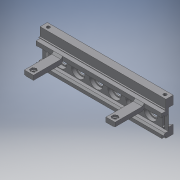
# Autodesk Inventor part: Case_top_back
Saved by Autodesk Inventor 2016 SP2 (Build 200236200, 236)
## iProperties
Created: 2018-06-26
Part Number: Case_top_back
Material: Generisch
Document SubType Name: Modeling
Designer: Nils
Density: 1 g/cm^3
Appearance: Vorgabe
Author: Nils
Autodesk Inventor part; units mm, degrees
ref_plane "YZ Plane" through (0, 0, 0) normal (1, 0, 0) x (0, 1, 0)
ref_plane "XZ Plane" through (0, 0, 0) normal (0, 1, 0) x (-1, 0, 0)
ref_plane "XY Plane" through (0, 0, 0) normal (0, 0, 1) x (1, 0, 0)
sketch "Skizze1" plane through (0, 0, 0) normal (1, 0, 0) x (0, 1, 0)
  line L0 (14.121, -6.5137) -> (22.121, -6.5137) projected
  line L1 (14.121, -15.8137) -> (14.121, -6.5137) projected
  line L2 (22.121, -6.5137) -> (22.121, -15.9372) projected
  line L3 (22.121, -34.3902) -> (22.121, -43.8137) projected
  line L4 (22.121, -43.8137) -> (14.121, -43.8137) projected
  line L5 (14.121, -38.3137) -> (14.121, -43.8137) projected
  line L6 (12.621, -15.8137) -> (14.121, -15.8137) projected
  line L7 (12.621, -15.8137) -> (12.621, -16.3137) projected
  line L8 (14.121, -17.8137) -> (12.621, -16.3137) projected
  line L9 (22.121, -15.9372) -> (22.121, -34.3902)
  line L10 (14.121, -43.8137) -> (14.121, -41.8137)
  line L11 (14.121, -41.8137) -> (9.621, -41.8137)
  line L12 (9.621, -41.8137) -> (9.621, -38.3137)
  line L13 (9.621, -38.3137) -> (11.421, -40.1137)
  line L14 (11.421, -40.1137) -> (13.221, -38.3137)
  line L15 (13.221, -38.3137) -> (16.691, -38.3137)
  line L16 (16.691, -38.3137) -> (16.691, -22.3437)
  line L17 (16.691, -22.3437) -> (13.221, -22.3437)
  line L18 (13.221, -22.3437) -> (11.421, -20.5437)
  line L19 (13.221, -22.3437) -> (15.7666, -22.3437) construction
  line L20 (11.421, -20.5437) -> (9.621, -22.3437)
  line L21 (9.621, -22.3437) -> (9.621, -17.8137)
  line L22 (9.621, -17.8137) -> (14.121, -17.8137)
  point P0 (0, 0)
  dimension "d0" = 2
  dimension "d1" = 4.5
  dimension "d2" = 3.5
  dimension "d3" = 3.47
  dimension "d4" = 15.97
  dimension "d5" = 1.8
  dimension "d6" = 45
  dimension "d7" = 135
  dimension "d8" = 4.53
  dimension "d9" = 1.8
  dimension "d10" = 4.5
  constraints: 28 end point, 7 perpendicular, 2 equal length, 2 vertical, 1 horizontal, 1 parallel, 1 point on line
  measures "d0" distance of L4.end L10.end
  measures "d1" distance of L10.end L11.end
  measures "d2" distance of L11.end L12.end
  measures "d3" distance of L14.end L15.end
  measures "d4" distance of L15.end L16.end
  measures "d5" horizontal distance of L12.end L13.end
  measures "d6" angle of L13 L12
  measures "d7" angle of L19 L18
  measures "d8" distance of L20.end L21.end
  measures "d9" horizontal distance of L18.end L17.end
  measures "d10" distance of L21.end L8.start
extrude "Extrusion1" add sketch "Skizze1" along normal blind 69.4
sketch "Skizze2" plane through (0, 22.121, -6.5137) normal (0, 1, 0) x (1, 0, 0)
  line L0 (128.7, 33.8232) -> (128.7, 3.4768) projected
  line L1 (0, 0) -> (138.8, 0) projected
  line L2 (10.1, 3.4768) -> (10.1, 33.8232) projected
  line L3 (0, 37.3) -> (138.8, 37.3) projected
  line L4 (0, 9.308) -> (0, 27.992)
  line L5 (0, 37.3) -> (0, 0) projected
  line L6 (138.8, 27.992) -> (128.7, 33.8232) projected
  line L7 (128.7, 3.4768) -> (138.8, 9.308) projected
  line L8 (138.8, 0) -> (138.8, 9.308) projected
  line L9 (0, 0) -> (0, 9.308) projected
  line L10 (0, 9.308) -> (10.1, 3.4768) projected
  line L11 (10.1, 33.8232) -> (0, 27.992) projected
  line L12 (0, 27.992) -> (0, 37.3) projected
  line L13 (138.8, 27.992) -> (138.8, 37.3) projected
  point P0 (0, -6.5137)
  constraints: 2 end point, 1 collinear
extrude "Extrusion2" cut sketch "Skizze2" against normal blind 5 contours L11 L2 L10 L4
sketch "Skizze3" plane through (0, 9.621, -22.3437) normal (0, -1, 0) x (1, 0, 0)
  line L0 (19.4, 2.53) -> (29.4, 2.53) projected
  line L1 (29.4, 2.53) -> (29.4, -2.47) projected
  line L2 (29.4, -2.47) -> (19.4, -2.47) projected
  line L3 (19.4, -2.47) -> (19.4, 2.53) projected
  point P0 (0, 22.3437)
extrude "Extrusion3" add sketch "Skizze3" along normal blind 32.25
chamfer "Fase1" distance 2.4 angle 45 1 edges at (24.4, 9.621, -24.8137)
chamfer "Fase2" distance 2 angle 45 1 edges at (24.4, 9.621, -19.8137)
sketch "Skizze4" plane through (29.4, -22.629, -24.8137) normal (0, 0, -1) x (-1, 0, 0)
  circle A0 centre (5, 5) radius 1.75
  line L0 (0, 0) -> (10, 0) projected
  line L1 (10, 30.25) -> (10, 0) projected
  point P0 (29.4, 22.629)
  point P1 (10, 32.25)
  dimension "d23" = 3.5
  dimension "d24" = 5
  dimension "d25" = 5
  constraints: 1 centre point
  measures "d23" diameter of A0
  measures "d24" distance from line of L0 A0.centre
  measures "d25" distance from line of L1 A0.centre
extrude "Extrusion4" cut sketch "Skizze4" against normal blind 32.25
sketch "Skizze6" plane through (0, 14.121, -6.5137) normal (0, 0, 1) x (1, 0, 0)
  circle A0 centre (5, 4) radius 1.75 projected
  point P0 (0, -14.121)
extrude "Extrusion5" cut sketch "Skizze6" against normal blind 34.75
sketch "Skizze7" plane through (0, 9.621, -22.3437) normal (0, -1, 0) x (1, 0, 0)
  line L0 (7.85, -1.42) -> (2.15, -1.42) projected
  line L1 (7.85, -4.22) -> (7.85, -1.42) projected
  line L2 (2.15, -4.22) -> (7.85, -4.22) projected
  line L3 (2.15, -1.42) -> (2.15, -4.22) projected
  point P0 (0, 22.3437)
extrude "Extrusion6" cut sketch "Skizze7" against normal blind 11.25
mirror "Spiegeln1" about plane through (69.4, 16.8296, -26.0997) normal (1, 0, 0) of "Extrusion6", "Extrusion5", "Extrusion4", "Extrusion3", "Extrusion2", "Extrusion1", "Fase2", "Fase1"
sketch "Skizze8" plane through (0, 22.121, -34.5057) normal (0, 1, 0) x (1, 0, 0)
  line L0 (134.8088, -12.162) -> (138.8, -12.162) construction
  line L1 (6.0088, -12.162) -> (6.0088, -10.742) construction
  line L2 (3.9912, -10.742) -> (3.9912, -12.162) construction
  line L3 (0, -12.162) -> (3.9912, -12.162) construction
  line L4 (0, -12.162) -> (0, 3.808) construction
  line L5 (6.0088, 3.808) -> (132.7912, 3.808) construction
  line L6 (138.8, -12.162) -> (138.8, 3.808) construction
  line L7 (6.0088, -12.162) -> (132.7912, -12.162) construction
  line L8 (134.8088, -7.942) -> (134.8088, 3.808) construction
  line L9 (132.7912, 3.808) -> (132.7912, -7.942) construction
  line L10 (138.8, -4.177) -> (0, -4.177) construction
  circle A0 centre (119.4, -4.177) radius 6
  circle A1 centre (99.4, -4.177) radius 6
  circle A2 centre (79.4, -4.177) radius 6
  circle A3 centre (59.4, -4.177) radius 6
  circle A4 centre (39.4, -4.177) radius 6
  circle A5 centre (19.4, -4.177) radius 6
  line L11 (0, 3.808) -> (3.9912, 3.808) projected
  line L12 (134.8088, 3.808) -> (138.8, 3.808) projected
  line L13 (132.7912, -7.942) -> (130.95, -7.942) projected
  line L14 (130.95, -7.942) -> (130.95, -10.742) projected
  line L15 (130.95, -10.742) -> (132.7912, -10.742) projected
  line L16 (132.7912, -10.742) -> (132.7912, -12.162) projected
  line L17 (6.0088, -10.742) -> (7.85, -10.742) projected
  line L18 (7.85, -10.742) -> (7.85, -7.942) projected
  line L19 (7.85, -7.942) -> (6.0088, -7.942) projected
  line L20 (6.0088, -7.942) -> (6.0088, 3.808) projected
  line L21 (3.9912, -7.942) -> (2.15, -7.942) projected
  line L22 (2.15, -7.942) -> (2.15, -10.742) projected
  line L23 (2.15, -10.742) -> (3.9912, -10.742) projected
  line L24 (3.9912, 3.808) -> (3.9912, -7.942) projected
  line L25 (134.8088, -12.162) -> (134.8088, -10.742) projected
  line L26 (134.8088, -10.742) -> (136.65, -10.742) projected
  line L27 (136.65, -10.742) -> (136.65, -7.942) projected
  line L28 (136.65, -7.942) -> (134.8088, -7.942) projected
  point P0 (0, -34.5057)
  dimension "d32" = 12
  dimension "d33" = 19.4
  dimension "d36" = 20
  constraints: 6 centre point, 2 end point, 2 midpoint, 1 horizontal, 1 point on line, 10 other
  measures "d32" diameter of A0
  measures "d33" distance from line of L6 A0.centre
  measures "d36" distance of A0.centre A1.centre
extrude "Extrusion7" cut sketch "Skizze8" against normal blind 5430
sketch "Skizze9" plane through (0, 16.691, -38.3137) normal (0, -1, 0) x (1, 0, 0)
  circle A0 centre (19.4, 7.985) radius 6 projected
  circle A1 centre (39.4, 7.985) radius 6 projected
  circle A2 centre (59.4, 7.985) radius 6 projected
  circle A3 centre (79.4, 7.985) radius 6 projected
  circle A4 centre (99.4, 7.985) radius 6 projected
  circle A5 centre (119.4, 7.985) radius 6 projected
  circle A6 centre (19.4, 7.985) radius 7.5
  circle A7 centre (39.4, 7.985) radius 7.5
  circle A8 centre (59.4, 7.985) radius 7.5
  circle A9 centre (79.4, 7.985) radius 7.5
  circle A10 centre (99.4, 7.985) radius 7.5
  circle A11 centre (119.4, 7.985) radius 7.5
  point P0 (0, 38.3137)
  dimension "d43" = 15
  dimension "d44" = 15
  dimension "d45" = 15
  dimension "d46" = 15
  dimension "d47" = 15
  dimension "d48" = 15
  constraints: 6 centre point, 6 coincident
  measures "d43" diameter of A6
  measures "d44" diameter of A7
  measures "d45" diameter of A8
  measures "d46" diameter of A9
  measures "d47" diameter of A10
  measures "d48" diameter of A11
extrude "Extrusion8" cut sketch "Skizze9" against normal blind 4
sketch "Skizze10" plane through (19.4, -22.629, -19.8137) normal (0, 0, 1) x (1, 0, 0)
  circle A0 centre (5, 5) radius 1.75 construction
  circle A1 centre (95, 5) radius 1.75 construction
  line L0 (2.15, 6.6454) -> (5, 8.2909)
  line L1 (5, 8.2909) -> (7.85, 6.6454)
  line L2 (7.85, 6.6454) -> (7.85, 3.3546)
  line L3 (7.85, 3.3546) -> (5, 1.7091)
  line L4 (5, 1.7091) -> (2.15, 3.3546)
  line L5 (2.15, 3.3546) -> (2.15, 6.6454)
  circle A2 centre (95, 5) radius 1.75 projected
  line L6 (92.15, 6.6454) -> (95, 8.2909)
  line L7 (95, 8.2909) -> (97.85, 6.6454)
  line L8 (97.85, 6.6454) -> (97.85, 3.3546)
  line L9 (97.85, 3.3546) -> (95, 1.7091)
  line L10 (95, 1.7091) -> (92.15, 3.3546)
  line L11 (92.15, 3.3546) -> (92.15, 6.6454)
  point P0 (-19.4, 22.629)
  dimension "d51" = 5.7
  dimension "d52" = 5.7
  constraints: 24 end point, 2 coincident, 2 vertical, 26 other
  measures "d51" distance between parallel lines of L2 L5
  measures "d52" distance between parallel lines of L8 L11
extrude "Extrusion9" cut sketch "Skizze10" against normal blind 2.2
